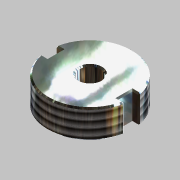
# Autodesk Inventor part: YTP-AP-E16-R1.0
Saved by Autodesk Inventor 2020.4 (Build 244396010, 396A)
## iProperties
RuleStatus: InUse
AfterDocNew0: iPropertyEnforcement
BeforeDocSave0: Materialprüfung
Created: 2021-08-29
Part Number: YTP-AP-E16-R1.0
Material: Allgemein
Document SubType Name: Modeling
Designer: Uwe Wieser
Mass: 0.0507797 g
Surface Area: 0.98294 cm^2
Volume: 0.0507797 cm^3
Density: 1 g/cm^3
Appearance: Chrom - poliert
Project: Airbrush
Description: Einstellschraube-Ventil
Werkstoff: 1.4301
Author: Uwe Wieser
Autodesk Inventor part; units mm, degrees
ref_plane "YZ Plane" through (0, 0, 0) normal (1, 0, 0) x (0, 1, 0)
ref_plane "XZ Plane" through (0, 0, 0) normal (0, 1, 0) x (-1, 0, 0)
ref_plane "XY Plane" through (0, 0, 0) normal (0, 0, 1) x (1, 0, 0)
sketch "Skizze1" plane through (0, 0, 0) normal (0, 0, 1) x (1, 0, 0)
  line L0 (-2.5, 0.5) -> (-2.5, -0.5)
  line L1 (2.5, 0.5) -> (2.5, -0.5)
  line L2 (-4.1413, 0) -> (4.1413, 0) projected
  line L3 (0, -4.2) -> (0, 4.2) projected
  circle A0 centre (0, 0) radius 0.75
  line L4 (-2.5, 0.5) -> (-2.958, 0.5)
  line L5 (-2.5, -0.5) -> (-2.958, -0.5)
  line L6 (2.5, -0.5) -> (2.958, -0.5)
  line L7 (2.5, 0.5) -> (2.958, 0.5)
  arc A1 (-2.958, -0.5) -> (2.958, -0.5) centre (0, 0) ccw
  arc A2 (2.958, 0.5) -> (-2.958, 0.5) centre (0, 0) ccw
  dimension "d0" = 1.5
  dimension "d8" = 5
  dimension "d9" = 3
  dimension "d10" = 3
  dimension "d11" = 0.458
  constraints: 12 end point, 4 point on circle, 3 centre point, 2 midpoint, 2 parallel, 2 point on line, 1 coincident, 1 horizontal, 2 other
  measures "d0" diameter of A0
  measures "d8" distance between parallel lines of L1 L0
  measures "d9" radius of A2
  measures "d10" radius of A1
  measures "d11" distance of L1.start L7.end
extrude "Extrusion2" add sketch "Skizze1" along normal mid plane 2 contours L4 A2 L3 A0 L2 L0 | L2 A0 L3 A1 L5 L0 | A2 L7 L1 L2 A0 L3 | A0 L2 L1 L6 A1 L3
chamfer "Fase1" distance 0.1 angle 45 22 edges at (-0.75, 0, 1) (0, 3, 1) (0, -3, 1) (0, -3, -1) (0, 3, -1) (-0.75, 0, -1) (-2.958, -0.5, 0) (-2.729, -0.5, -1) (-2.5, 0, -1) (-2.5, 0, 1) (-2.729, -0.5, 1) (-2.729, 0.5, -1) (-2.729, 0.5, 1) (-2.958, 0.5, 0) (2.958, -0.5, 0) (2.958, 0.5, 0) (2.729, 0.5, -1) (2.729, 0.5, 1) (2.5, 0, -1) (2.729, -0.5, -1) (2.729, -0.5, 1) (2.5, 0, 1)
thread "Gewinde2" size "M6x0.5" class "6g" standard "ISO Metric profile" length 10
